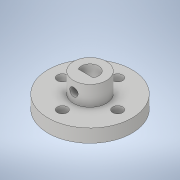
# Autodesk Inventor part: Horn_Attachment
Saved by Autodesk Inventor 2022 (Build 260153000, 153)
## iProperties
Created: 2020-10-11
Part Number: Horn_Attachment
Material: Generic
Document SubType Name: Modeling
Designer: Mlees
Density: 1 g/cm^3
Appearance: Default
Author: Mlees
Autodesk Inventor part; units mm, degrees
ref_plane "YZ Plane" through (0, 0, 0) normal (1, 0, 0) x (0, 1, 0)
ref_plane "XZ Plane" through (0, 0, 0) normal (0, 1, 0) x (-1, 0, 0)
sketch "Sketch1" plane through (0, 0, 0) normal (0, 1, 0) x (-1, 0, 0)
  circle A0 centre (0, 0) radius 12.7
  dimension "d0" = 25.4
  constraints: 1 centre point, 1 coincident
  measures "d0" diameter of A0
extrude "Extrusion1" add sketch "Sketch1" along normal blind 4
sketch "Sketch2" plane through (0, 4, 0) normal (0, 1, 0) x (1, 0, 0)
  circle A0 centre (0, 8.382) radius 1.524
  circle A1 centre (0, 0) radius 12.7 projected
  circle A2 centre (-8.382, 0) radius 1.524
  circle A3 centre (0, -8.382) radius 1.524
  circle A4 centre (8.382, 0) radius 1.524
  dimension "d7" = 360
  constraints: 4 centre point, 9 other
extrude "Extrusion2" cut sketch "Sketch2" along normal mid plane 8 contours A0 | A2 | A3 | A4
sketch "Sketch10" plane through (0, 0, 0) normal (0, -1, 0) x (1, 0, 0)
  circle A0 centre (0, 0) radius 12.7 projected
  circle A1 centre (0, 0) radius 3.5
  dimension "d49" = 7
  constraints: 1 centre point, 1 coincident
  measures "d49" diameter of A1
extrude "Extrusion9" cut sketch "Sketch10" against normal blind 2 contours A1
sketch "Sketch11" plane through (0, 4, 0) normal (0, 1, 0) x (1, 0, 0)
  circle A0 centre (0, 0) radius 3.5 projected
  circle A1 centre (0, 0) radius 5
  circle A2 centre (0, 0) radius 2.625
  dimension "d52" = 10
  dimension "d53" = 5.25
  constraints: 2 centre point, 2 coincident
  measures "d52" diameter of A1
  measures "d53" diameter of A2
extrude "Extrusion10" add sketch "Sketch11" along normal blind 6 contours A0 | A1
sketch "Sketch12" plane through (0, 10, 0) normal (0, 1, 0) x (1, 0, 0)
  line L0 (0, -1.3125) -> (-2.2733, -1.3125)
  circle A0 centre (0, 0) radius 2.625 projected
  arc A1 (-2.2733, -1.3125) -> (2.2733, -1.3125) centre (0, 0) ccw
  line L1 (0, -1.3125) -> (2.2733, -1.3125)
  dimension "d56" = 1.3125
  constraints: 4 end point, 4 point on circle, 1 centre point, 1 concentric, 1 horizontal, 1 point on line
  measures "d56" distance of point (0, 0) L0.start
extrude "Extrusion11" add sketch "Sketch12" against normal up to surface (6 mm away) contours L1 A0 L0 picked at (1.3942, -1.4755)
ref_plane "Work Plane1" through (0, 4, 5) normal (0, 0, -1) x (-1, 0, 0)
sketch "Sketch13" plane through (0, 4, 5) normal (0, 0, -1) x (-1, 0, 0)
  line L0 (5, 6) -> (-5, 6) projected
  circle A0 centre (0, 3) radius 1.25
  point P0 (0, -4)
  dimension "d60" = 2.5
  constraints: 1 centre point
  measures "d60" diameter of A0
extrude "Extrusion12" cut sketch "Sketch13" along normal up to surface (3.6875 mm away)
body "Solid1"
